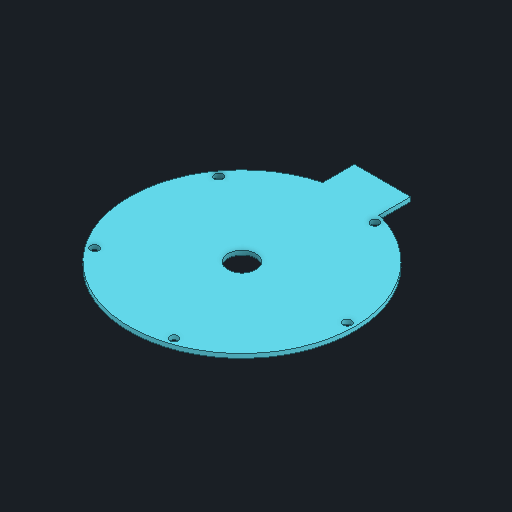
# Autodesk Inventor part: femur_motor_steel
Saved by Autodesk Inventor 2026 (Build 300175000, 175)
## iProperties
Created: 2026-04-24
Part Number: femur_motor_steel
Material: Сталь
Document SubType Name: Modeling
Designer: user
Density: 7.85 g/cm^3
Appearance: Серо-синий
Mass: 557.654 g
Surface Area: 499.57 cm^2
Volume: 71.0387 cm^3
Author: user
Autodesk Inventor part; units mm, degrees
ref_plane "YZ Plane" through (0, 0, 0) normal (1, 0, 0) x (0, 1, 0)
ref_plane "XZ Plane" through (0, 0, 0) normal (0, 1, 0) x (-1, 0, 0)
ref_plane "XY Plane" through (0, 0, 0) normal (0, 0, 1) x (1, 0, 0)
sketch "Эскиз1" plane through (0, 0, 0) normal (0, 1, 0) x (-1, 0, 0)
  circle A0 centre (-168.9344, 188.7011) radius 75 construction
  circle A1 centre (-108.2116, 232.7209) radius 3.05
  circle A2 centre (-192.0353, 260.0548) radius 3.05
  circle A3 centre (-243.9343, 188.7803) radius 3.05
  circle A4 centre (-192.186, 117.3964) radius 3.05
  circle A5 centre (-108.3047, 144.5532) radius 3.05
  arc A6 (-148.9344, 111.2415) -> (-188.9344, 111.2415) centre (-168.9344, 188.7011) ccw
  line L0 (-188.9344, 88.7011) -> (-148.9344, 88.7011)
  line L1 (-148.9344, 88.7011) -> (-148.9344, 111.2415)
  line L2 (-188.9344, 111.2415) -> (-188.9344, 88.7011)
  circle A7 centre (-168.9344, 188.7011) radius 10
  point P0 (0, 0)
  dimension "d4" = 150
  dimension "d5" = 6.1
  dimension "d8" = 360
  dimension "d10" = 160
  dimension "d13" = 20
  dimension "d14" = 40
  dimension "d15" = 100
  dimension "d16" = 20
  constraints: 7 centre point, 6 end point, 2 coincident, 2 point on circle, 1 horizontal, 1 parallel, 1 perpendicular, 15 other
  measures "d5" diameter of A1
  measures "d10" diameter of A6
  measures "d13" distance from line of point (-168.934, 188.701) L1
  measures "d14" distance between parallel lines of L1 L2
  measures "d15" distance from line of point (-168.934, 188.701) L0
  measures "d16" diameter of A7
extrude "Выдавливание1" add sketch "Эскиз1" along normal blind 3
equation "\"d5\" = d_main_screw_holes"
equation "\"d13\" = 0.5 * hight_coxa"
equation "\"d14\" = hight_coxa"
equation "\"d15\" = length_coxa"
equation "\"d16\" = d_main_shaft"
equation "\"d2\" = thickness_steel"
equation "\"tolerance_plazma\" = 0.1"
equation "\"thickness_steel\" = 3"
equation "\"d_main_screw_holes\" = 6.1"
equation "\"d_main_shaft\" = 20"
equation "\"thickness_profile_tibea\" = 3"
equation "\"hight_shaft_shift\" = 37"
equation "\"thickness_profile_femur\" = 3"
equation "\"width_shaft_shift\" = 35"
equation "\"width_flattened_surface\" = 12"
equation "\"length_coxa\" = 100"
equation "\"hight_coxa\" = 40"
